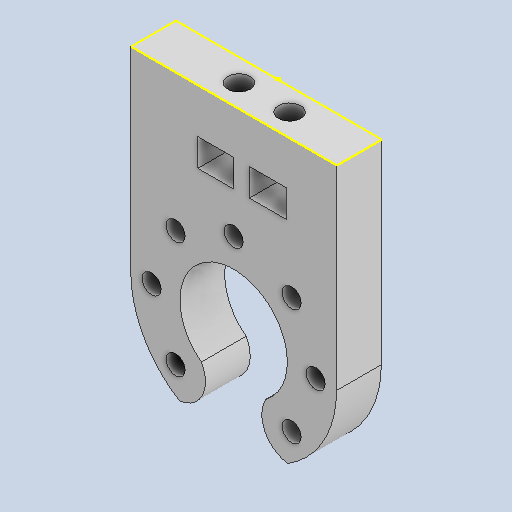
# Autodesk Inventor part: 0904_foot_adt
Saved by Autodesk Inventor 2024.3 (Build 283343000, 343)
## iProperties
Created: 2024-09-04
Part Number: 0904_foot_adt
Material: 일반
Document SubType Name: Modeling
Designer: gretc
Density: 1 g/cm^3
Appearance: 기본값
Author: gretc
Autodesk Inventor part; units mm, degrees
ref_plane "YZ Plane" through (0, 0, 0) normal (1, 0, 0) x (0, 1, 0)
ref_plane "XZ Plane" through (0, 0, 0) normal (0, 1, 0) x (-1, 0, 0)
ref_plane "XY Plane" through (0, 0, 0) normal (0, 0, 1) x (1, 0, 0)
sketch "스케치1" plane through (0, 0, 0) normal (0, 0, 1) x (1, 0, 0)
  circle A0 centre (0, 0) radius 13.8 projected
  circle A1 centre (0, 0) radius 7.2 projected
  circle A2 centre (0, -11) radius 1.2812 projected
  circle A3 centre (-7.7782, -7.7782) radius 1.2812 projected
  circle A4 centre (-11, 0) radius 1.2812 projected
  circle A5 centre (-7.7782, 7.7782) radius 1.2812 projected
  circle A6 centre (0, 11) radius 1.2812 projected
  circle A7 centre (7.7782, 7.7782) radius 1.2812 projected
  circle A8 centre (11, 0) radius 1.2812 projected
  circle A9 centre (7.7782, -7.7782) radius 1.2812 projected
  circle A10 centre (7.7782, -7.7782) radius 4
  circle A11 centre (-7.7782, -7.7782) radius 4
  line L0 (13.8, 0) -> (-13.8, 0)
  line L1 (-13.8, 0) -> (-13.8, 26.193)
  line L2 (-13.8, 26.193) -> (13.8, 26.193)
  line L3 (13.8, 26.193) -> (13.8, 0)
  arc A12 (-19.5808, 6.2636) -> (-20.1, 4.5766) centre (-17.1, 4.5766) ccw projected
  line L4 (-20.1, -39.6766) -> (-20.1, 4.5766) projected
  arc A13 (-20.1, -39.6766) -> (-19.5808, -41.3636) centre (-17.1, -39.6766) ccw projected
  line L5 (-15.8929, -46.7869) -> (-19.5808, -41.3636) projected
  arc A14 (-15.8929, -46.7869) -> (-13.4121, -48.1) centre (-13.4121, -45.1) ccw projected
  line L6 (13.4121, -48.1) -> (-13.4121, -48.1) projected
  arc A15 (13.4121, -48.1) -> (15.8929, -46.7869) centre (13.4121, -45.1) ccw projected
  line L7 (19.5808, -41.3636) -> (15.8929, -46.7869) projected
  arc A16 (19.5808, -41.3636) -> (20.1, -39.6766) centre (17.1, -39.6766) ccw projected
  line L8 (20.1, 4.5766) -> (20.1, -39.6766) projected
  arc A17 (20.1, 4.5766) -> (19.5808, 6.2636) centre (17.1, 4.5766) ccw projected
  line L9 (15.5953, 12.1246) -> (19.5808, 6.2636) projected
  arc A18 (15.5953, 12.1246) -> (13.9414, 13) centre (13.9414, 11) ccw projected
  line L10 (7.65, 13) -> (13.9414, 13) projected
  arc A19 (9.15, 11.5) -> (7.65, 13) centre (7.65, 11.5) ccw projected
  line L11 (9.15, 11.5) -> (9.15, 10) projected
  arc A20 (9.15, 10) -> (11.5, 7.65) centre (11.5, 10) ccw projected
  line L12 (11.5, 7.65) -> (13.5, 7.65) projected
  arc A21 (14.5, 6.65) -> (13.5, 7.65) centre (13.5, 6.65) ccw projected
  line L13 (14.5, 6.65) -> (14.5, -36.15) projected
  arc A22 (13.5, -37.15) -> (14.5, -36.15) centre (13.5, -36.15) ccw projected
  line L14 (13.5, -37.15) -> (11.5, -37.15) projected
  arc A23 (11.5, -37.15) -> (9.15, -39.5) centre (11.5, -39.5) ccw projected
  line L15 (9.15, -39.5) -> (9.15, -41.5) projected
  arc A24 (8.15, -42.5) -> (9.15, -41.5) centre (8.15, -41.5) ccw projected
  line L16 (8.15, -42.5) -> (-8.15, -42.5) projected
  arc A25 (-9.15, -41.5) -> (-8.15, -42.5) centre (-8.15, -41.5) ccw projected
  line L17 (-9.15, -41.5) -> (-9.15, -39.5) projected
  arc A26 (-9.15, -39.5) -> (-11.5, -37.15) centre (-11.5, -39.5) ccw projected
  line L18 (-11.5, -37.15) -> (-13.5, -37.15) projected
  arc A27 (-14.5, -36.15) -> (-13.5, -37.15) centre (-13.5, -36.15) ccw projected
  line L19 (-14.5, -36.15) -> (-14.5, 6.65) projected
  arc A28 (-13.5, 7.65) -> (-14.5, 6.65) centre (-13.5, 6.65) ccw projected
  line L20 (-13.5, 7.65) -> (-11.5, 7.65) projected
  arc A29 (-11.5, 7.65) -> (-9.15, 10) centre (-11.5, 10) ccw projected
  line L21 (-9.15, 10) -> (-9.15, 11.5) projected
  arc A30 (-7.65, 13) -> (-9.15, 11.5) centre (-7.65, 11.5) ccw projected
  line L22 (-13.9414, 13) -> (-7.65, 13) projected
  arc A31 (-13.9414, 13) -> (-15.5953, 12.1246) centre (-13.9414, 11) ccw projected
  line L23 (-19.5808, 6.2636) -> (-15.5953, 12.1246) projected
  circle A32 centre (17.3, 4) radius 1.35 projected
  circle A33 centre (17.3, -18) radius 1.35 projected
  circle A34 centre (11, -45.3) radius 1.35 projected
  circle A35 centre (-17.3, 4) radius 1.35 projected
  circle A36 centre (-17.3, -18) radius 1.35 projected
  circle A37 centre (-11, -45.3) radius 1.35 projected
  circle A38 centre (17.3, -40) radius 1.35 projected
  circle A39 centre (-17.3, -40) radius 1.35 projected
  line L24 (15, 14.5) -> (-15, 14.5) projected
  point P0 (0, 0)
  point P1 (4.3283, -5.7538)
  point P2 (7.2486, -11.743)
  point P3 (-7.2486, -11.743)
  point P4 (-4.3283, -5.7538)
  dimension "d0" = 8
  dimension "d1" = 8
  dimension "d2" = 27.6
  dimension "d3" = 26.193
  dimension "d4" = 14.5
  constraints: 8 end point, 2 centre point, 2 coincident, 2 parallel, 1 horizontal, 1 perpendicular, 2 other
  measures "d0" diameter of A10
  measures "d1" diameter of A11
  measures "d2" distance of L1.end L2.end
  measures "d3" distance between parallel lines of L2 L0
  measures "d4" distance between parallel lines of L24 L0
extrude "돌출1" add sketch "스케치1" along normal blind 6 contours L0 A8 A1 A4 A0 A29 L21 L11 A20 | A0 A10 A1 L0 A8 | A0 A20 L12 A21 L3 | A20 L11 A0 | A0 L11 A19 L10 L3 A21 L12 A20 | A0 A10 A1 | A0 L21 A30 L22 L1 L24 L3 L10 A19 L11 | L21 A29 A0 | A0 A29 L20 A28 L1 L22 A30 L21 | A0 A11 A1 | L24 L1 L2 L3 | A0 L1 A28 L20 A29 | A0 L0 A4 A1 A11
sketch "스케치2" plane through (-13.8, 26.193, 0) normal (0, 1, 0) x (1, 0, 0)
  line L0 (27.6, 0) -> (0, 0) projected
  line L1 (0, 0) -> (0, -6) projected
  line L2 (27.6, -6) -> (0, -6) projected
  line L3 (27.6, 0) -> (27.6, -6) projected
  point P0 (13.8, 0)
sketch "스케치3" plane through (-13.8, 26.193, 0) normal (0, 1, 0) x (1, 0, 0)
  line L0 (13.8, 0) -> (13.8, -6)
  line L1 (21, -6) -> (6.6, -6) projected
  line L2 (27.6, 0) -> (27.6, -6) projected
  line L3 (27.6, -6) -> (18.3, -6)
  line L4 (18.3, -6) -> (18.3, 0)
  line L5 (17.5782, 0) -> (21.0486, 0) projected
  line L6 (18.3, -6) -> (11.5187, -6)
  line L7 (21, 0) -> (6.6, 0) projected
  line L8 (11.5187, 0) -> (11.5187, -6)
  line L9 (27.6, -6) -> (27.6, -3.263)
  line L10 (0, 0) -> (0, -6) projected
  line L11 (0, -3) -> (27.6, -3)
  circle A0 centre (11.5187, -3) radius 1.5
  circle A1 centre (18.3, -3) radius 1.5
  point P0 (9.4717, -6)
  point P1 (18.1283, -6)
  point P2 (18.1283, 0)
  point P3 (9.4717, 0)
  dimension "d7" = 9.3
  dimension "d8" = 3
  dimension "d9" = 3
  constraints: 14 end point, 7 point on line, 5 midpoint, 2 centre point, 2 perpendicular
  measures "d7" distance of L2.end L3.end
  measures "d8" diameter of A0
  measures "d9" diameter of A1
extrude "돌출2" cut sketch "스케치3" against normal blind 6 contours A0 L8 L11 | L11 L8 A0 | A1 L4 L11 | L11 L4 A1 | L8 L11 A0 | L8 A0 L11 | L11 A1 L4 | L4 A1 L11
sketch "스케치4" plane through (0, 0, 6) normal (0, 0, 1) x (1, 0, 0)
  line L0 (-3.7813, 20.193) -> (-0.7813, 20.193) projected
  line L1 (3, 20.193) -> (6, 20.193) projected
  line L2 (-3.7813, 26.193) -> (-3.7813, 20.193) projected
  line L3 (-0.7813, 26.193) -> (-0.7813, 20.193) projected
  line L4 (3, 26.193) -> (3, 20.193) projected
  line L5 (6, 26.193) -> (6, 20.193) projected
  line L6 (-4.7987, 20.193) -> (0.0243, 20.193)
  line L7 (0.0243, 20.193) -> (0.0243, 16.5095)
  line L8 (0.0243, 16.5095) -> (-4.7987, 16.5095)
  line L9 (-4.7987, 16.5095) -> (-4.7987, 20.193)
  line L10 (2.1205, 16.5095) -> (7.0764, 16.5095)
  line L11 (7.0764, 16.5095) -> (7.0764, 20.193)
  line L12 (7.0764, 20.193) -> (2.1205, 20.193)
  line L13 (2.1205, 20.193) -> (2.1205, 16.5095)
  point P0 (0, 0)
  constraints: 16 end point, 4 parallel, 2 horizontal, 2 perpendicular
extrude "돌출3" cut sketch "스케치4" against normal blind 6
